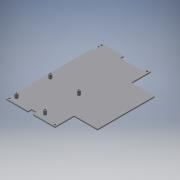
# Autodesk Inventor part: Part53
Saved by Autodesk Inventor 2016 (Build 200138000, 138)
## iProperties
Created: 2015-11-07
Part Number: Part53
Material: Generic
Document SubType Name: Modeling
Designer: Jufo
Density: 1 g/cm^3
Appearance: Default
Author: Jufo
Autodesk Inventor part; units mm, degrees
ref_plane "YZ Plane" through (0, 0, 0) normal (1, 0, 0) x (0, 1, 0)
ref_plane "XZ Plane" through (0, 0, 0) normal (0, 1, 0) x (-1, 0, 0)
ref_plane "XY Plane" through (0, 0, 0) normal (0, 0, 1) x (1, 0, 0)
sketch "Sketch1" plane through (0, 0, 0) normal (0, 1, 0) x (-1, 0, 0)
  line L0 (49.278, 4.7758) -> (49.278, -28.2242)
  line L1 (49.278, -28.2242) -> (87.278, -28.2242)
  line L2 (87.278, -28.2242) -> (87.278, -22.2242)
  line L3 (87.278, -22.2242) -> (95.278, -22.2242)
  line L4 (95.278, -22.2242) -> (95.278, -28.2242)
  line L5 (95.278, 135.7758) -> (95.278, 129.7758)
  line L6 (95.278, 129.7758) -> (87.278, 129.7758)
  line L7 (87.278, 129.7758) -> (87.278, 135.7758)
  line L8 (87.278, 135.7758) -> (49.278, 135.7758)
  line L9 (49.278, 135.7758) -> (49.278, 102.7758)
  line L10 (49.278, 4.7758) -> (9.278, 4.7758)
  line L11 (9.278, 4.7758) -> (9.278, 102.7758)
  line L12 (9.278, 102.7758) -> (49.278, 102.7758)
  line L13 (94.278, 130.7758) -> (94.278, 136.7758)
  line L14 (48.278, 136.7758) -> (134.278, 136.7758)
  line L15 (134.278, -29.2242) -> (48.278, -29.2242)
  line L16 (94.278, -29.2242) -> (94.278, -23.2242)
  line L17 (94.278, -23.2242) -> (88.278, -23.2242)
  line L18 (88.278, -23.2242) -> (88.278, -29.2242)
  line L19 (48.278, -29.2242) -> (48.278, 3.7758)
  line L20 (48.278, 3.7758) -> (24.278, 3.7758)
  line L21 (24.278, 103.7758) -> (48.278, 103.7758)
  line L22 (48.278, 103.7758) -> (48.278, 136.7758)
  line L23 (88.278, 136.7758) -> (88.278, 130.7758)
  line L24 (24.278, 3.7758) -> (8.278, 3.7758)
  line L25 (24.278, 103.7758) -> (8.278, 103.7758)
  line L26 (8.278, 103.7758) -> (8.278, 3.7758)
  line L27 (94.278, 130.7758) -> (88.278, 130.7758)
  line L28 (134.278, -29.2242) -> (134.278, 136.7758)
  line L29 (95.278, 135.7758) -> (134.278, 135.7758)
  line L30 (95.278, -28.2242) -> (134.278, -28.2242)
  line L31 (134.278, 135.7758) -> (133.278, 135.7758)
  line L32 (133.278, 135.7758) -> (133.278, -28.2242)
  line L33 (133.278, -28.2242) -> (134.278, -28.2242)
  line L34 (134.278, -28.2242) -> (134.278, 135.7758)
  point P0 (0, 0)
  point P1 (0, 0)
  dimension "d0" = 1
  dimension "d4" = 1
  dimension "d5" = 1
  dimension "d6" = 1
  dimension "d7" = 1
  dimension "d8" = 1
  dimension "d10" = 1
  dimension "d11" = 1
  dimension "d12" = 1
  dimension "d13" = 1
  dimension "d14" = 1
  dimension "d15" = 1
  dimension "d16" = 6
  dimension "d17" = 0
  dimension "d18" = 0
  dimension "d25" = 1
  dimension "d75" = 164
  dimension "d76" = 164
  dimension "d77" = 166
  dimension "d79" = 33
  dimension "d82" = 33
  constraints: 70 end point, 13 perpendicular, 5 point on line, 4 horizontal, 1 parallel
  measures "d0" distance from line of L5.start L13
  measures "d4" distance from line of L3.end L16
  measures "d5" distance between parallel lines of L3 L17
  measures "d6" distance between parallel lines of L18 L2
  measures "d7" distance between parallel lines of L19 L0
  measures "d8" distance between parallel lines of L10 L20
  measures "d10" distance between parallel lines of L15 L1
  measures "d11" distance from line of L21 L9.end
  measures "d12" distance between parallel lines of L9 L22
  measures "d13" distance between parallel lines of L23 L7
  measures "d14" distance between parallel lines of L14 L8
  measures "d15" distance between parallel lines of L6 L27
  measures "d16" distance of L23.start L23.end
  measures "d17" distance from line of L14 L13.end
  measures "d18" distance from line of L14 L23.start
  measures "d25" distance of L29.end L31.end
  measures "d75" distance between parallel lines of L29 L30
  measures "d76" distance between parallel lines of L1 L8
  measures "d77" distance between parallel lines of L14 L15
  measures "d79" distance of L8.end L9.end
  measures "d82" distance of L0.start L0.end
extrude "Extrusion2" add sketch "Sketch1" along normal blind 2 contours L10 L11 L12 L9 L8 L7 L6 L5 L29 L32 L30 L4 L3 L2 L1 L0
sketch "Sketch2" plane through (0, 2, 0) normal (0, 1, 0) x (1, 0, 0)
  circle A0 centre (-52.278, 25.2242) radius 1.5
  line L0 (-49.278, -4.7758) -> (-49.278, 28.2242) projected
  line L1 (-49.278, 28.2242) -> (-87.278, 28.2242) projected
  line L2 (-87.278, 22.2242) -> (-95.278, 22.2242) projected
  line L3 (-91.278, 22.2242) -> (-91.278, -30.1136)
  circle A1 centre (-130.278, 25.2242) radius 1.5
  line L4 (-9.278, -102.7758) -> (-9.278, -4.7758) projected
  line L5 (-9.278, -53.7758) -> (-80.3163, -53.7758)
  circle A2 centre (-52.278, -132.7758) radius 1.5
  circle A3 centre (-130.278, -132.7758) radius 1.5
  point P0 (0, 0)
  dimension "d26" = 3
  dimension "d27" = 3
  dimension "d28" = 3
  constraints: 4 centre point, 4 end point, 3 symmetric about line, 2 midpoint, 1 horizontal, 1 vertical, 3 other
  measures "d26" diameter of A0
  measures "d27" distance from line of A0.centre L0
  measures "d28" distance from line of L1 A0.centre
extrude "Extrusion3" cut sketch "Sketch2" against normal blind 10
sketch "Sketch3" plane through (0, 2, 0) normal (0, 1, 0) x (1, 0, 0)
  circle A0 centre (-76.278, -67.7758) radius 1.25
  circle A1 centre (-76.278, -67.7758) radius 1.25
  circle A2 centre (-76.278, -125.7758) radius 1.25
  circle A3 centre (-76.278, -125.7758) radius 1.25
  circle A4 centre (-125.278, -67.7758) radius 1.25
  circle A5 centre (-125.278, -67.7758) radius 1.25
  circle A6 centre (-125.278, -125.7758) radius 1.25
  circle A7 centre (-125.278, -125.7758) radius 1.25
  line L0 (-87.278, -135.7758) -> (-49.278, -135.7758) projected
  line L1 (-133.278, 28.2242) -> (-133.278, -135.7758) projected
  circle A8 centre (-76.278, -67.7758) radius 2.5
  circle A9 centre (-76.278, -125.7758) radius 2.5
  circle A10 centre (-125.278, -67.7758) radius 2.5
  circle A11 centre (-125.278, -125.7758) radius 2.5
  point P0 (0, 0)
  point P1 (40, -28)
  dimension "d31" = 49
  dimension "d32" = 58
  dimension "d33" = 49
  dimension "d34" = 58
  dimension "d35" = 10
  dimension "d36" = 10
  dimension "d37" = 8
  dimension "d38" = 8
  dimension "d70" = 5
  dimension "d71" = 5
  dimension "d72" = 5
  dimension "d73" = 5
  constraints: 12 centre point, 8 coincident
  measures "d31" distance of A5.centre A1.centre
  measures "d32" distance of A3.centre A1.centre
  measures "d33" distance of A7.centre A3.centre
  measures "d34" distance of A7.centre A5.centre
  measures "d35" distance from line of L0 A6.centre
  measures "d36" distance from line of L0 A3.centre
  measures "d37" distance from line of L1 A6.centre
  measures "d38" distance from line of L1 A4.centre
  measures "d70" diameter of A8
  measures "d71" diameter of A9
  measures "d72" diameter of A10
  measures "d73" diameter of A11
extrude "Extrusion4" add sketch "Sketch3" along normal blind 7
sketch "Sketch6" plane through (0, 2, 0) normal (0, 1, 0) x (1, 0, 0)
  line L0 (-133.278, 28.2242) -> (-133.278, -135.7758) projected
  line L1 (-133.278, 28.2242) -> (-133.278, 21.2242)
  line L2 (-133.278, 21.2242) -> (-129.278, 21.2242)
  line L3 (-129.278, 21.2242) -> (-129.278, 12.2242)
  line L4 (-129.278, 12.2242) -> (-133.278, 12.2242)
  line L5 (-133.278, 21.2242) -> (-133.278, 12.2242)
  line L6 (-133.278, -135.7758) -> (-133.278, -128.7758)
  line L7 (-133.278, -128.7758) -> (-129.278, -128.7758)
  line L8 (-129.278, -128.7758) -> (-129.278, -119.7758)
  line L9 (-129.278, -119.7758) -> (-133.278, -119.7758)
  line L10 (-133.278, -128.7758) -> (-133.278, -119.7758)
  point P0 (0, 0)
  dimension "d63" = 7
  dimension "d64" = 4
  dimension "d65" = 9
  dimension "d66" = 7
  dimension "d67" = 9
  dimension "d83" = 4
  constraints: 20 end point, 5 perpendicular, 4 point on line, 2 collinear, 1 vertical
  measures "d63" distance of L0.start L1.end
  measures "d64" distance of L1.end L2.end
  measures "d65" distance of L2.end L3.end
  measures "d66" distance of L0.end L6.end
  measures "d67" distance of L7.end L8.end
  measures "d83" distance between parallel lines of L0 L8
extrude "Extrusion7" cut sketch "Sketch6" against normal blind 10
sketch "Sketch7" plane through (0, 2, 0) normal (0, 1, 0) x (1, 0, 0)
  line L0 (-49.278, -4.7758) -> (-49.278, 28.2242) projected
  line L1 (-49.278, 28.2242) -> (-87.278, 28.2242) projected
  line L2 (-87.278, 28.2242) -> (-87.278, 22.2242) projected
  line L3 (-9.278, -102.7758) -> (-9.278, -4.7758) projected
  line L4 (-9.278, -4.7758) -> (-49.278, -4.7758) projected
  line L5 (-49.278, -102.7758) -> (-9.278, -102.7758) projected
  line L6 (-87.278, 28.2242) -> (-87.278, 13.2242)
  line L7 (-87.278, 13.2242) -> (-57.278, 13.2242)
  line L8 (-57.278, 13.2242) -> (-57.278, 28.2242)
  line L9 (-49.278, 28.2242) -> (-87.278, 28.2242) projected
  point P0 (0, 0)
  dimension "d94" = 15
  constraints: 6 end point, 2 perpendicular, 1 point on line, 1 vertical
  measures "d94" distance of L1.end L6.end
extrude "Extrusion8" cut sketch "Sketch7" against normal blind 10
equation "\"d36\" = d35"
equation "\"d38\" = d37"
body "Solid2"
